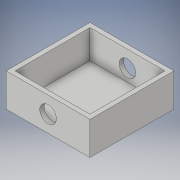
# Autodesk Inventor part: Caja_ampli_antena
Saved by Autodesk Inventor 2019.3 (Build 233278000, 278)
## iProperties
Created: 2019-04-13
Part Number: Caja_ampli_antena
Material: Generic
Document SubType Name: Modeling
Designer: garri
Density: 1 g/cm^3
Appearance: Default
Author: garri
## iProperties of the stored document Caja_ampli_antena_3DPrint.ipt
Created: 2019-04-13
Part Number: Caja_ampli_antena_3DPrint
Material: Generic
Document SubType Name: Modeling
Designer: garri
Density: 1 g/cm^3
Appearance: Default
Author: garri
Autodesk Inventor part; units mm, degrees
ref_plane "YZ Plane" through (0, 0, 0) normal (1, 0, 0) x (0, 1, 0)
ref_plane "XZ Plane" through (0, 0, 0) normal (0, 1, 0) x (-1, 0, 0)
ref_plane "XY Plane" through (0, 0, 0) normal (0, 0, 1) x (1, 0, 0)
sketch "Sketch1" plane through (0, 0, 0) normal (0, 1, 0) x (-1, 0, 0)
  line L0 (76, 0.0718) -> (0, 0.0718)
  line L1 (0, 0.0718) -> (0, -75.9282)
  line L2 (0, -75.9282) -> (76, -75.9282)
  line L3 (76, -75.9282) -> (76, 0.0718)
  point P0 (0, 0)
  dimension "d0" = 76
  dimension "d1" = 76
  constraints: 8 end point, 2 parallel, 1 horizontal, 1 perpendicular
  measures "d0" distance of L1.end L2.end
  measures "d1" distance of L0.end L1.end
extrude "Extrusion1" add sketch "Sketch1" along normal blind 30
shell "Shell1" thickness 4 removed faces 1 at (-50.6667, 30, -25.2616)
sketch "Sketch2" plane through (-76, 0, 0.0718) normal (0, 0, 1) x (1, 0, 0)
  line L0 (0, 30) -> (76, 30) projected
  line L1 (38, 30) -> (38, 0)
  line L2 (0, 0) -> (76, 0) projected
  line L3 (0, 0) -> (0, 30) projected
  line L4 (0, 15) -> (76, 15)
  line L5 (76, 0) -> (76, 30) projected
  circle A0 centre (38, 15) radius 7.5
  dimension "d5" = 15
  constraints: 5 midpoint, 4 end point, 1 centre point
  measures "d5" diameter of A0
hole "Hole1" at (-38, 15, 0.0718) direction (0, 0, -1) diameter 15 end through all
body "Solid1"
